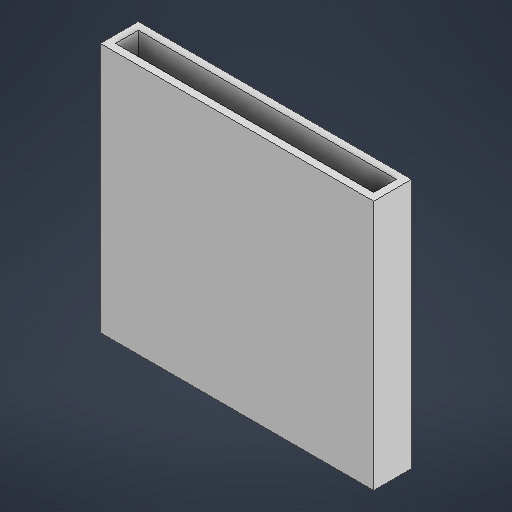
# Autodesk Inventor part: sing_cell_bottom_case_alternate
Saved by Autodesk Inventor 2026 (Build 300175050, 175E)
## iProperties
Created: 2025-06-19
Part Number: sing_cell_bottom_case_alternate
Material: Generic
Document SubType Name: Modeling
Designer: hamth
Density: 1 g/cm^3
Appearance: Default
Author: hamth
Autodesk Inventor part; units mm, degrees
ref_plane "YZ Plane" through (0, 0, 0) normal (1, 0, 0) x (0, 1, 0)
ref_plane "XZ Plane" through (0, 0, 0) normal (0, 1, 0) x (-1, 0, 0)
ref_plane "XY Plane" through (0, 0, 0) normal (0, 0, 1) x (1, 0, 0)
sketch "Sketch1" plane through (0, 0, 0) normal (0, 1, 0) x (-1, 0, 0)
  line L0 (43.1683, -15.7294) -> (-71.1317, -15.7294)
  line L1 (-71.1317, -15.7294) -> (-71.1317, 0.1456)
  line L2 (-71.1317, 0.1456) -> (43.1683, 0.1456)
  line L3 (43.1683, 0.1456) -> (43.1683, -15.7294)
  point P0 (0, 0)
  dimension "d0" = 114.3
  dimension "d1" = 15.875
  constraints: 8 end point, 2 parallel, 1 horizontal, 1 perpendicular
  measures "d0" distance of L0.start L0.end
  measures "d1" distance of L2.end L0.start
extrude "Extrusion1" add sketch "Sketch1" along normal blind 3.175
sketch "Sketch6" plane through (0, 3.175, 0) normal (0, 1, 0) x (1, 0, 0)
  line L0 (71.1317, 15.7294) -> (-43.1683, 15.7294) projected
  line L1 (-43.1683, 15.7294) -> (71.1317, 15.7294)
  line L2 (71.1317, 15.7294) -> (71.1317, 12.5544)
  line L3 (71.1317, 12.5544) -> (-43.1683, 12.5544)
  line L4 (-43.1683, 12.5544) -> (-43.1683, 15.7294)
  point P0 (0, 0)
  dimension "d33" = 3.175
  dimension "d34" = 114.3
  constraints: 8 end point, 2 parallel, 1 perpendicular, 1 point on line
  measures "d33" distance of L1.end L2.end
  measures "d34" distance of L2.end L3.end
extrude "Extrusion2" add sketch "Sketch6" along normal blind 101.6
sketch "Sketch9" plane through (0, 3.175, 0) normal (0, 1, 0) x (1, 0, 0)
  line L0 (-43.1683, -0.1456) -> (71.1317, -0.1456) projected
  line L1 (-43.1683, -0.1456) -> (71.1317, -0.1456)
  line L2 (71.1317, -0.1456) -> (71.1317, 3.0294)
  line L3 (71.1317, 3.0294) -> (-43.1683, 3.0294)
  line L4 (-43.1683, 3.0294) -> (-43.1683, -0.1456)
  point P0 (0, 0)
  dimension "d41" = 3.175
  dimension "d42" = 114.3
  constraints: 8 end point, 2 parallel, 1 perpendicular, 1 point on line
  measures "d41" distance of L1.end L2.end
  measures "d42" distance of L2.end L3.end
extrude "Extrusion3" add sketch "Sketch9" along normal blind 101.6
sketch "Sketch11" plane through (0, 3.175, 0) normal (0, 1, 0) x (1, 0, 0)
  line L0 (-43.1683, 12.5544) -> (71.1317, 12.5544) projected
  line L1 (-43.1683, 12.5544) -> (-39.9933, 12.5544)
  line L2 (-39.9933, 12.5544) -> (-39.9933, 3.0294)
  line L3 (-39.9933, 3.0294) -> (-43.1683, 3.0294)
  line L4 (-43.1683, 3.0294) -> (-43.1683, 12.5544)
  point P0 (0, 0)
  dimension "d45" = 3.175
  dimension "d46" = 9.525
  constraints: 8 end point, 2 parallel, 1 perpendicular, 1 point on line
  measures "d45" distance of L2.end L3.end
  measures "d46" distance of L1.end L2.end
extrude "Extrusion4" add sketch "Sketch11" along normal blind 101.6
sketch "Sketch13" plane through (0, 3.175, 0) normal (0, 1, 0) x (1, 0, 0)
  line L0 (71.1317, 12.5544) -> (-39.9933, 12.5544) projected
  line L1 (71.1317, 12.5544) -> (67.9567, 12.5544)
  line L2 (67.9567, 12.5544) -> (67.9567, 3.0294)
  line L3 (67.9567, 3.0294) -> (71.1317, 3.0294)
  line L4 (71.1317, 3.0294) -> (71.1317, 12.5544)
  point P0 (0, 0)
  dimension "d51" = 3.175
  dimension "d52" = 9.525
  constraints: 8 end point, 2 parallel, 1 perpendicular, 1 point on line
  measures "d51" distance of L2.end L3.end
  measures "d52" distance of L1.end L2.end
extrude "Extrusion5" add sketch "Sketch13" along normal blind 101.6
sketch "Sketch14" plane through (0, 3.175, 0) normal (0, 1, 0) x (1, 0, 0)
  line L0 (67.9567, 12.5544) -> (-39.9933, 12.5544) projected
  line L1 (-39.9933, 12.5544) -> (67.9567, 12.5544)
  line L2 (67.9567, 12.5544) -> (67.9567, 9.3794)
  line L3 (67.9567, 9.3794) -> (-39.9933, 9.3794)
  line L4 (-39.9933, 9.3794) -> (-39.9933, 12.5544)
  point P0 (0, 0)
  dimension "d55" = 3.175
  dimension "d56" = 107.95
  constraints: 8 end point, 2 parallel, 1 perpendicular, 1 point on line
  measures "d55" distance of L1.end L2.end
  measures "d56" distance of L2.end L3.end
extrude "Extrusion6" add sketch "Sketch14" along normal blind 3.175
sketch "Sketch15" plane through (0, 3.175, 0) normal (0, 1, 0) x (1, 0, 0)
  line L0 (67.9567, 3.0294) -> (-39.9933, 3.0294) projected
  line L1 (-39.9933, 3.0294) -> (67.9567, 3.0294)
  line L2 (67.9567, 3.0294) -> (67.9567, 6.2044)
  line L3 (67.9567, 6.2044) -> (-39.9933, 6.2044)
  line L4 (-39.9933, 6.2044) -> (-39.9933, 3.0294)
  point P0 (0, 0)
  dimension "d59" = 3.175
  dimension "d60" = 107.95
  constraints: 8 end point, 2 parallel, 1 perpendicular, 1 point on line
  measures "d59" distance of L1.end L2.end
  measures "d60" distance of L2.end L3.end
extrude "Extrusion7" add sketch "Sketch15" along normal blind 3.175
sketch "Sketch17" plane through (0, 3.175, 0) normal (0, 1, 0) x (1, 0, 0)
  line L0 (67.9567, 9.3794) -> (-39.9933, 9.3794) projected
  line L1 (-39.9933, 9.3794) -> (-36.8183, 9.3794)
  line L2 (-36.8183, 9.3794) -> (-36.8183, 6.2044)
  line L3 (-36.8183, 6.2044) -> (-39.9933, 6.2044)
  line L4 (-39.9933, 6.2044) -> (-39.9933, 9.3794)
  point P0 (0, 0)
  dimension "d64" = 3.175
  dimension "d65" = 3.175
  constraints: 8 end point, 2 parallel, 1 perpendicular, 1 point on line
  measures "d64" distance of L2.end L3.end
  measures "d65" distance of L1.end L2.end
extrude "Extrusion8" add sketch "Sketch17" along normal blind 3.175
sketch "Sketch18" plane through (0, 3.175, 0) normal (0, 1, 0) x (1, 0, 0)
  line L0 (-36.8183, 9.3794) -> (67.9567, 9.3794) projected
  line L1 (67.9567, 9.3794) -> (64.7817, 9.3794)
  line L2 (64.7817, 9.3794) -> (64.7817, 6.2044)
  line L3 (64.7817, 6.2044) -> (67.9567, 6.2044)
  line L4 (67.9567, 6.2044) -> (67.9567, 9.3794)
  point P0 (0, 0)
  dimension "d68" = 3.175
  dimension "d69" = 3.175
  constraints: 8 end point, 2 parallel, 1 perpendicular, 1 point on line
  measures "d68" distance of L2.end L3.end
  measures "d69" distance of L1.end L2.end
extrude "Extrusion9" add sketch "Sketch18" along normal blind 3.175
sketch "Sketch20" plane through (0, 104.775, 0) normal (0, 1, 0) x (1, 0, 0)
  line L0 (-43.1683, -0.1456) -> (71.1317, -0.1456) projected
  line L1 (-43.1683, -0.1456) -> (-43.1683, 7.7919)
  line L2 (-43.1683, 15.7294) -> (-43.1683, -0.1456) projected
  line L3 (-43.1683, 7.7919) -> (13.9817, 7.7919)
  point P0 (0, 0)
  dimension "d79" = 7.9375
  dimension "d80" = 57.15
  constraints: 4 end point, 1 midpoint, 1 perpendicular
  measures "d79" distance of L0.start L1.end
  measures "d80" distance of L1.end L3.end
hole "Hole6" at (13.9817, 104.775, -7.7919) direction (0, -1, 0) diameter 3.175 end through all
body "Solid1"
